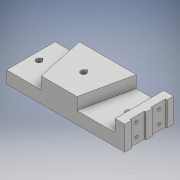
# Autodesk Inventor part: Part02
Saved by Autodesk Inventor 2018 (Build 220112000, 112)
## iProperties
Created: 2019-02-06
Part Number: Part02
Material: Generic
Document SubType Name: Modeling
Designer: JARVIS
Density: 1 g/cm^3
Appearance: Default
Author: JARVIS
Autodesk Inventor part; units mm, degrees
ref_plane "YZ Plane" through (0, 0, 0) normal (1, 0, 0) x (0, 1, 0)
ref_plane "XZ Plane" through (0, 0, 0) normal (0, 1, 0) x (-1, 0, 0)
ref_plane "XY Plane" through (0, 0, 0) normal (0, 0, 1) x (1, 0, 0)
sketch "Sketch1" plane through (0, 0, 0) normal (0, 0, 1) x (1, 0, 0)
  line L0 (-32.5, 15) -> (32.5, 15)
  line L1 (32.5, 15) -> (32.5, -15)
  line L2 (32.5, -15) -> (-32.5, -15)
  line L3 (-32.5, -15) -> (-32.5, 15)
  point P0 (0, 0)
  point P1 (0, 15)
  point P2 (32.5, 0)
  dimension "d0" = 65
  dimension "d1" = 30
  constraints: 8 end point, 2 midpoint, 2 parallel, 1 horizontal, 1 horizontal alignment, 1 perpendicular, 1 vertical alignment
  measures "d0" distance of L0.start L0.end
  measures "d1" distance of L2.end L0.start
extrude "Extrusion1" add sketch "Sketch1" along normal blind 7.5
sketch "Sketch2" plane through (0, 0, 7.5) normal (0, 0, 1) x (1, 0, 0)
  line L0 (32.5, 15) -> (-32.5, 15) projected
  line L1 (-17.5, 15) -> (-11, -15)
  line L2 (-32.5, -15) -> (32.5, -15) projected
  line L3 (11, -15) -> (17.5, 15)
  line L4 (-17.5, 15) -> (17.5, 15)
  line L5 (-11, -15) -> (11, -15)
  point P0 (0, 0)
  dimension "d4" = 22
  dimension "d5" = 35
  dimension "d6" = 15
  dimension "d7" = 21.5
  constraints: 8 end point, 3 point on line, 2 collinear
  measures "d4" distance of L3.start L1.end
  measures "d5" distance of L3.end L1.start
  measures "d6" distance of L0.end L1.start
  measures "d7" distance of L1.end L2.start
extrude "Extrusion2" add sketch "Sketch2" along normal blind 7.5
sketch "Sketch3" plane through (0, 0, 0) normal (0, 0, -1) x (-1, 0, 0)
  arc A0 (-28.7374, 1.2374) -> (-26.2626, 1.2374) centre (-27.5, 0) ccw
  arc A1 (26.2626, 1.2374) -> (28.7374, 1.2374) centre (27.5, 0) ccw
  arc A2 (-1.2374, 1.2374) -> (1.2374, 1.2374) centre (0, 0) ccw
  line L0 (32.5, -15) -> (32.5, 15) projected
  line L1 (-32.5, 15) -> (-32.5, -15) projected
  line L2 (-26.2626, 1.2374) -> (-27.5, 2.4749)
  line L3 (-27.5, 2.4749) -> (-28.7374, 1.2374)
  line L4 (-1.2374, 1.2374) -> (0, 2.4749)
  line L5 (0, 2.4749) -> (1.2374, 1.2374)
  line L6 (26.2626, 1.2374) -> (27.5, 2.4749)
  line L7 (27.5, 2.4749) -> (28.7374, 1.2374)
  dimension "d10" = 5
  dimension "d11" = 5
  dimension "d12" = 3.5
  dimension "d39" = 90
  dimension "d40" = 90
  dimension "d41" = 90
  constraints: 13 end point, 7 point on circle, 3 centre point, 3 horizontal alignment, 3 tangent, 3 vertical alignment, 2 equal radius, 2 perpendicular, 1 coincident, 1 point on line
  measures "d10" distance from line of L0 A1.centre
  measures "d11" distance from line of L1 A0.centre
  measures "d12" diameter of A1
  measures "d39" angle of L5 L4
  measures "d40" angle of L2 L3
  measures "d41" angle of L7 L6
extrude "Extrusion3" cut sketch "Sketch3" against normal through all
sketch "Sketch4" plane through (0, 0, 0) normal (0, 0, -1) x (-1, 0, 0)
  circle A0 centre (-27.5, 0) radius 1.75 projected
  line L0 (-24.5, 1.7321) -> (-24.5, -1.7321)
  line L1 (-24.5, -1.7321) -> (-27.5, -3.4641)
  line L2 (-27.5, -3.4641) -> (-30.5, -1.7321)
  line L3 (-30.5, -1.7321) -> (-30.5, 1.7321)
  line L4 (-30.5, 1.7321) -> (-27.5, 3.4641)
  line L5 (-27.5, 3.4641) -> (-24.5, 1.7321)
  line L6 (0, 3.4641) -> (3, 1.7321)
  line L7 (3, 1.7321) -> (3, -1.7321)
  line L8 (3, -1.7321) -> (0, -3.4641)
  line L9 (0, -3.4641) -> (-3, -1.7321)
  line L10 (-3, -1.7321) -> (-3, 1.7321)
  line L11 (-3, 1.7321) -> (0, 3.4641)
  circle A1 centre (27.5, 0) radius 1.75 projected
  line L12 (30.5, 1.7321) -> (30.5, -1.7321)
  line L13 (30.5, -1.7321) -> (27.5, -3.4641)
  line L14 (27.5, -3.4641) -> (24.5, -1.7321)
  line L15 (24.5, -1.7321) -> (24.5, 1.7321)
  line L16 (24.5, 1.7321) -> (27.5, 3.4641)
  line L17 (27.5, 3.4641) -> (30.5, 1.7321)
  circle A2 centre (0, 0) radius 1.75 projected
  dimension "d15" = 6
  dimension "d16" = 6
  dimension "d17" = 6
  constraints: 36 end point, 3 coincident, 3 vertical, 39 other
  measures "d15" distance between parallel lines of L11 L8
  measures "d16" distance between parallel lines of L17 L14
  measures "d17" distance between parallel lines of L2 L5
extrude "Extrusion4" cut sketch "Sketch4" against normal blind 3
sketch "Sketch5" plane through (32.5, -15, 0) normal (1, 0, 0) x (0, 0, -1)
  line L0 (0, 30) -> (0, 0) projected
  line L1 (0, 30) -> (-7.5, 30) projected
  line L2 (-7.5, 0) -> (-7.5, 30) projected
  line L3 (0, 0) -> (-7.5, 0) projected
  point P0 (0, 15)
extrude "Extrusion5" add sketch "Sketch5" along normal blind 2
sketch "Sketch6" plane through (34.5, -15, 0) normal (1, 0, 0) x (0, 0, -1)
  line L0 (-7.5, 30) -> (-15, 30) projected
  line L1 (-15, 30) -> (0, 30)
  line L2 (0, 30) -> (0, 0)
  line L3 (0, 0) -> (-15, 0)
  line L4 (-15, 0) -> (-15, 30)
  line L5 (0, 0) -> (0, 30) projected
  line L6 (-7.5, 0) -> (0, 0) projected
  point P0 (0, 15)
  point P1 (0, 15)
  point P2 (0, 15)
  point P3 (-3.75, 0)
  constraints: 8 end point, 4 midpoint, 2 parallel, 1 coincident, 1 horizontal, 1 horizontal alignment, 1 perpendicular
extrude "Extrusion6" add sketch "Sketch6" along normal blind 5
sketch "Sketch7" plane through (39.5, -15, 0) normal (1, 0, 0) x (0, 0, -1)
  line L0 (-7.5, 30) -> (-7.5, 0) projected
  arc A0 (-12.2071, 22.7071) -> (-10.7929, 22.7071) centre (-11.5, 22) ccw
  arc A1 (-4.2071, 22.7071) -> (-2.7929, 22.7071) centre (-3.5, 22) ccw
  arc A2 (-12.2071, 8.7071) -> (-10.7929, 8.7071) centre (-11.5, 8) ccw
  arc A3 (-4.2071, 8.7071) -> (-2.7929, 8.7071) centre (-3.5, 8) ccw
  line L1 (-15, 0) -> (0, 0) projected
  line L2 (-15, 30) -> (-15, 0) projected
  line L3 (-15, 0) -> (0, 0) projected
  line L4 (0, 0) -> (0, 30) projected
  line L5 (0, 30) -> (-15, 30) projected
  line L6 (-12.2071, 22.7071) -> (-11.5, 23.4142)
  line L7 (-11.5, 23.4142) -> (-10.7929, 22.7071)
  line L8 (-4.2071, 22.7071) -> (-3.5, 23.4142)
  line L9 (-3.5, 23.4142) -> (-2.7929, 22.7071)
  line L10 (-4.2071, 8.7071) -> (-3.5, 9.4142)
  line L11 (-3.5, 9.4142) -> (-2.7929, 8.7071)
  line L12 (-12.2071, 8.7071) -> (-11.5, 9.4142)
  line L13 (-11.5, 9.4142) -> (-10.7929, 8.7071)
  point P0 (0, 15)
  dimension "d26" = 2
  dimension "d27" = 14
  dimension "d28" = 8
  dimension "d29" = 8
  dimension "d30" = 3.5
  dimension "d42" = 90
  dimension "d43" = 90
  dimension "d44" = 90
  dimension "d45" = 90
  constraints: 16 end point, 8 point on circle, 7 tangent, 6 vertical alignment, 4 centre point, 3 equal radius, 2 horizontal alignment, 1 perpendicular
  measures "d26" diameter of A1
  measures "d27" distance of A2.centre A0.centre
  measures "d28" distance from line of L1 A2.centre
  measures "d29" distance of A1.centre A0.centre
  measures "d30" distance from line of A0.centre L2
  measures "d42" angle of L7 L6
  measures "d43" angle of L9 L8
  measures "d44" angle of L11 L10
  measures "d45" angle of L13 L12
extrude "Extrusion7" cut sketch "Sketch7" against normal blind 5 contours L6 L7 A0 | L8 L9 A1 | L12 L13 A2 | L10 L11 A3
sketch "Sketch8" plane through (39.5, -15, 0) normal (1, 0, 0) x (0, 0, -1)
  line L0 (-7.5, 30) -> (-15, 30) projected
  line L1 (-15, 30) -> (0, 30)
  line L2 (0, 30) -> (0, 26)
  line L3 (0, 26) -> (-15, 26)
  line L4 (-15, 26) -> (-15, 30)
  line L5 (-15, 30) -> (-15, 0) projected
  line L6 (0, 0) -> (0, 30) projected
  line L7 (-15, 17) -> (0, 17)
  line L8 (0, 17) -> (0, 13)
  line L9 (0, 13) -> (-15, 13)
  line L10 (-15, 13) -> (-15, 17)
  line L11 (-15, 4) -> (0, 4)
  line L12 (0, 4) -> (0, 0)
  line L13 (0, 0) -> (-15, 0)
  line L14 (-15, 0) -> (-15, 4)
  line L15 (-15, 0) -> (0, 0) projected
  point P0 (0, 15)
  point P1 (-7.5, 0)
  point P2 (-7.5, 0)
  dimension "d33" = 4
  dimension "d34" = 4
  dimension "d35" = 4
  dimension "d36" = 2
  constraints: 24 end point, 6 parallel, 4 point on line, 3 horizontal, 3 perpendicular, 2 midpoint, 1 coincident
  measures "d33" distance between parallel lines of L1 L3
  measures "d34" distance between parallel lines of L9 L7
  measures "d35" distance between parallel lines of L13 L11
  measures "d36" distance from line of point (0, 15) L9
extrude "Extrusion8" add sketch "Sketch8" along normal blind 1 contours L1 L2 L3 L4 L0 | L7 L6 L9 L5 | L11 L6 L13 L5
equation "\"d11\" = d10"
body "Solid1"
